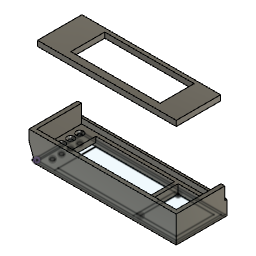
OLED0.91_border_face v0 (Autodesk Fusion 360 design; units mm, degrees)
Autodesk Fusion 360 part; units mm, degrees
note: some values were not read from the file. Set by a fixed rule: which face or edge a step refers to.
sketch "Sketch1" plane through (0, 0, 0) normal (0, 0, 1) x (1, 0, 0)
  line L0 (0, 0) -> (39, 0)
  line L1 (39, 0) -> (39, 12.5)
  line L2 (39, 12.5) -> (0, 12.5)
  line L3 (0, 12.5) -> (0, 0)
  circle A0 centre (2, 10) radius 0.5
  circle A1 centre (2, 7.46) radius 0.5
  circle A2 centre (2, 4.92) radius 0.5
  circle A3 centre (2, 2.38) radius 0.5
  line L4 (-0.6, -0.6) -> (39.6, -0.6)
  line L5 (39.6, -0.6) -> (39.6, 13.1)
  line L6 (39.6, 13.1) -> (-0.6, 13.1)
  line L7 (-0.6, 13.1) -> (-0.6, -0.6)
  line L8 (5, 1) -> (38, 1)
  line L9 (38, 1) -> (38, 11.5)
  line L10 (38, 11.5) -> (5, 11.5)
  line L11 (5, 11.5) -> (5, 1)
  line L12 (27, 1) -> (27, 11.5)
  line L13 (28, 1) -> (28, 11.5)
  line L14 (5, 1) -> (5, 0)
  line L15 (27, 1) -> (27, 0)
  line L16 (0.4, 13.1) -> (0.4, -0.6)
  line L17 (0, 12.5) -> (-0.6, 12.5)
  line L18 (39, 12.5) -> (39.6, 12.5)
  dimension "d1" = 39
  dimension "d2" = 12.5
  dimension "d3" = 1
  dimension "d4" = 2
  dimension "d5" = 2.5
  dimension "d8" = 0
  dimension "d9" = -7.62
  dimension "d10" = 0.6
  dimension "d12" = 5
  dimension "d18" = 1
  dimension "d19" = 1
  dimension "d20" = 1
  dimension "d21" = 11
  dimension "d22" = 1
  dimension "d28" = 1
  constraint horizontal L0
  constraint vertical L1
  constraint horizontal L2
  constraint vertical L3
  constraint coincident L0.start L3.end
  constraint parallel L0 L8
  constraint parallel L1 L9
  constraint parallel L2 L10
  constraint parallel L3 L11
  constraint coincident L11.start L10
  constraint coincident L8.start L11.end
  constraint coincident L10.end L11.start
  constraint coincident L8 L12.start
  constraint coincident L10 L12.end
  constraint perpendicular L10 L12
  constraint coincident L0 L14.end
  constraint perpendicular L0 L14
  constraint coincident L0 L15.end
  constraint perpendicular L0 L15
  constraint perpendicular L6 L16
  constraint coincident L6 L16.start
  constraint coincident L4 L16.end
  constraint coincident L7 L17.end
  constraint perpendicular L7 L17
  constraint coincident L5 L18.end
  constraint perpendicular L5 L18
  measures "d1" distance of L0.start L0.end
  measures "d2" distance of L0.start L2.end
  measures "d3" diameter of A0
  measures "d4" distance of L3 A0.centre
  measures "d5" distance of L2 A0.centre
  measures "d12" distance of L3 L11
  measures "d18" distance of L1 L9
  measures "d19" distance of L0 L8
  measures "d20" distance of L2 L10
  measures "d21" distance of L9 L12
  measures "d28" distance of L7 L16
extrude "Extrude1" add sketch "Sketch1" along normal blind 2.5 contours L0 L8 L14 L15 | L0 L1 L4 L5 L16 L18 | L0 L1 L2 L8 L9 L10 L11 L14 L15 L16 | L0 L3 L4 L7 L16 L17 | L0 L2 L3 L16 | L2 L5 L6 L16 L18 | L2 L6 L7 L16 L17 makes body 1
extrude "Extrude2" add sketch "Sketch1" along normal blind 5 from surface at 2.5 contours L0 L1 L4 L5 L16 L18 | L0 L3 L4 L7 L16 L17 | L2 L5 L6 L16 L18 | L2 L6 L7 L16 L17 bodies 1
extrude "Extrude3" add sketch "Sketch1" along normal blind 2.5 contours L8 L10 L12 L13 bodies 1
extrude "Extrude4" cut sketch "Sketch1" against normal blind 1.5 from surface at 2.5 contours L0 L8 L14 L15 bodies 1
extrude "Extrude5" cut sketch "Sketch1" along normal blind 0.5 contours L0 L3 L4 L7 L16 L17 | L0 L2 L3 L16 | L2 L6 L7 L16 L17 bodies 1
chamfer "Chamfer1" distance 1 angle 45 1 edges at (5, 6.25, 0) on bodies 1
chamfer "Chamfer3" distance 0.5 angle 45 4 edges at (1.5338, 2.5608, 0) (1.5338, 5.1008, 0) (1.5338, 7.6408, 0) (1.5338, 10.1808, 0) on bodies 1
chamfer "Chamfer4" distance 0.5 angle 45 4 edges at (1.5338, 10.1808, 2.5) (1.5338, 7.6408, 2.5) (1.5338, 5.1008, 2.5) (1.5338, 2.5608, 2.5) on bodies 1
extrude "Extrude7" cut sketch "Sketch1" against normal blind 3.5 from surface at 7.5 contours L2 L5 L6 L16 L18 | L2 L6 L7 L16 L17 bodies 1
move_face "OffsetFaces1" offset 0.5 3 faces at (26.5333, -0.6, 2.6667) (39.6, 3.7667, 3.8333) (-0.6, 3.7667, 4) on bodies 1
draft "Draft2" angle 70 neutral plane through (0.4, 0, 0) pull (-1, 0, 0) 1 faces at (-0.6, 8.3667, 0.5) on bodies 1
ref_plane "WorkPlane1" through (19.5, 5.7, 27.5) normal (0, 0, 1) x (1, 0, 0)
sketch "Sketch2" plane through (19.5, 5.7, 27.5) normal (0, 0, 1) x (1, 0, 0)
  line L0 (20.6, 6.8) -> (19.5, 6.8)
  line L1 (19.5, 6.8) -> (19.5, -5.7)
  line L2 (19.5, -5.7) -> (-19.5, -5.7)
  line L3 (-19.5, -5.7) -> (-19.5, 6.8)
  line L4 (-19.5, 6.8) -> (-20.6, 6.8)
  line L5 (-20.6, 6.8) -> (-20.6, -6.8)
  line L6 (-20.6, -6.8) -> (20.6, -6.8)
  line L7 (20.6, -6.8) -> (20.6, 6.8)
  line L8 (-19.5, 6.8) -> (19.5, 6.8)
  line L9 (19.5, 6.8) -> (19.5, -5.7)
  line L10 (19.5, -5.7) -> (-19.5, -5.7)
  line L11 (-19.5, -5.7) -> (-19.5, 6.8)
  line L12 (-19.5, 5.8) -> (19.5, 5.8)
  line L13 (-12, -5.7) -> (-12, 6.8)
  line L14 (19.5, -3.7) -> (-19.5, -3.7)
  line L15 (13, 6.8) -> (13, -5.7)
  point P0 (13, -3.7)
  point P1 (-12, -3.7)
  point P2 (-12, 5.8)
  point P3 (13, 5.8)
  dimension "d53" = 1
  dimension "d54" = 7.5
  dimension "d55" = 2
  dimension "d56" = 6.5
  constraint horizontal L8
  constraint vertical L9
  constraint horizontal L10
  constraint vertical L11
  constraint coincident L1.end L2.start
  constraint coincident L3.end L4.start
  constraint coincident L14 P0
  constraint coincident L15 P0
  constraint coincident L13 P1
  constraint coincident L14 P1
  constraint coincident L12 P2
  constraint coincident L13 P2
  constraint coincident L15 P3
  constraint coincident L12 P3
extrude "Extrude8" add sketch "Sketch2" along normal blind 1.5 separate body contours L1 L8 L9 L12 L15 | L1 L9 L12 L14 L15 | L8 L12 L13 L15 | L1 L2 L9 L10 L14 L15 | L3 L8 L11 L12 L13 | L2 L10 L13 L14 L15 | L3 L11 L12 L13 L14 | L2 L3 L10 L11 L13 L14 makes body 2
move_face "OffsetFaces2" offset -0.1 9 faces at (0, 11.8333, 28) (0, 5.1667, 28) (0, 0.6667, 28) (5, 0, 28.5) (24.1667, 0, 28.5) (36.8333, 0, 28.5) (39, 12.1667, 28) (39, 1.3333, 28) (39, 8.3333, 28) on bodies 2
